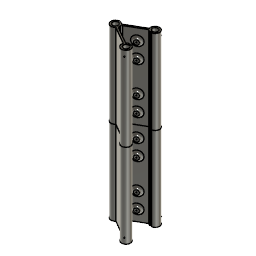
casomira-semafor-dlouhý (Autodesk Fusion 360 design; units mm, degrees)
Autodesk Fusion 360 part; units mm, degrees
other "Base Mesh Feature1" in component "part_object_id_3"
other "Base Mesh Feature1'" in component "part_object_id_2"
other "Base Mesh Feature1''" in component "part_object_id_1"
sketch "Sketch1" plane through (0, 0, 0) normal (0, 0, 1) x (1, 0, 0)
  circle A0 centre (69.45, 162.2) radius 5
  arc A1 (69.4, 161.6) -> (69.6, 161.6) centre (69.5, 162.4) ccw
  arc A2 (69.4, 161.6) -> (69.6, 161.6) centre (69.5, 162.3) ccw
  circle A3 centre (114.45, 188.2) radius 5
  circle A4 centre (114.45, 136.2003) radius 5
  line L0 (115.95, 142.25) -> (115.95, 182.2)
  line L1 (106.8955, 185.5676) -> (75.5037, 167.43)
  line L2 (75.5037, 156.97) -> (109.5697, 137.2876)
  line L3 (112.95, 142.25) -> (112.95, 182.2)
  line L4 (108.3963, 182.97) -> (77.0045, 164.8324)
  line L5 (77.0045, 159.5676) -> (108.3963, 141.4303)
  arc A5 (75.5037, 167.43) -> (75.5037, 156.97) centre (69.45, 162.2) ccw
  arc A6 (77.0045, 159.5676) -> (77.0045, 164.8324) centre (69.45, 162.2) ccw
  line L6 (114.45, 182.2) -> (112.95, 182.2)
  line L7 (114.45, 182.2) -> (115.95, 182.2)
  line L8 (114.45, 142.25) -> (112.95, 142.25)
  line L9 (114.45, 142.25) -> (115.95, 142.25)
  arc A7 (108.3963, 182.97) -> (112.95, 180.3419) centre (114.45, 188.2) ccw
  arc A8 (115.95, 180.3419) -> (106.8955, 185.5676) centre (114.45, 188.2) ccw
  arc A9 (106.8955, 138.8327) -> (115.95, 144.0584) centre (114.45, 136.2003) ccw
  arc A10 (112.95, 144.0584) -> (108.3963, 141.4303) centre (114.45, 136.2003) ccw
  line L10 (115.95, 182.2) -> (112.95, 182.2)
  line L11 (112.95, 182.2) -> (112.95, 142.25)
  line L12 (112.95, 142.25) -> (115.95, 142.25)
  line L13 (115.95, 142.25) -> (115.95, 182.2)
  dimension "d1" = 10
  dimension "d2" = 16
  dimension "d3" = 10
  dimension "d4" = 16
  dimension "d5" = 51.971
  dimension "d6" = 10
  dimension "d7" = 16
  constraint concentric A0 A5
  constraint concentric A3 A7
  constraint concentric A4 A9
  constraint concentric A5 A6
  constraint coincident A4 L2.end
  constraint perpendicular L3 L6
  constraint perpendicular L0 L7
  constraint perpendicular L3 L8
  constraint perpendicular L0 L9
  constraint coincident L2 A9.start
  constraint coincident L0 A8.start
  constraint concentric A7 A8
  constraint coincident L3 A7.end
  constraint coincident L0 A9.end
  constraint concentric A9 A10
  constraint coincident L3 A10.start
  constraint horizontal L10
  constraint vertical L11
  constraint horizontal L12
  constraint vertical L13
  measures "d1" diameter of A0
  measures "d2" diameter of A5
  measures "d3" diameter of A3
  measures "d4" diameter of A7
  measures "d5" distance of A0.centre A4.centre
  measures "d6" diameter of A4
  measures "d7" diameter of A9
sketch "Sketch2" plane through (0, 0, 0) normal (0, 1, 0) x (1, 0, 0)
extrude "Extrude1" add sketch "Sketch1" along normal blind 150 contours L0 L1 L2 L3 L4 L5 A5 A6 L6 L7 L8 L9 A7 A8 A9 A10 L10 L11 L12 L13 makes body 1
sketch "Sketch3" plane through (0, 0, 150) normal (0, 0, 1) x (-1, 0, 0)
  circle A0 centre (-114.45, -136.2003) radius 5
  circle A1 centre (-69.45, -162.2) radius 5
  circle A2 centre (-114.45, -188.2) radius 5
  arc A3 (-112.95, -144.0584) -> (-108.3963, -141.4303) centre (-114.45, -136.2003) ccw
  line L0 (-108.3963, -141.4303) -> (-77.0045, -159.5676)
  arc A4 (-77.0045, -159.5676) -> (-77.0045, -164.8324) centre (-69.45, -162.2) ccw
  line L1 (-77.0045, -164.8324) -> (-108.3963, -182.97)
  arc A5 (-108.3963, -182.97) -> (-112.95, -180.3419) centre (-114.45, -188.2) ccw
  line L2 (-112.95, -180.3419) -> (-112.95, -182.2)
  line L3 (-112.95, -182.2) -> (-115.95, -182.2)
  line L4 (-115.95, -182.2) -> (-115.95, -180.3419)
  arc A6 (-115.95, -180.3419) -> (-106.8955, -185.5676) centre (-114.45, -188.2) ccw
  line L5 (-106.8955, -185.5676) -> (-75.5037, -167.43)
  arc A7 (-75.5037, -167.43) -> (-75.5037, -156.97) centre (-69.45, -162.2) ccw
  line L6 (-75.5037, -156.97) -> (-106.8955, -138.8327)
  arc A8 (-106.8955, -138.8327) -> (-115.95, -144.0584) centre (-114.45, -136.2003) ccw
  line L7 (-115.95, -144.0584) -> (-115.95, -142.25)
  line L8 (-115.95, -142.25) -> (-112.95, -142.25)
  line L9 (-112.95, -142.25) -> (-112.95, -144.0584)
  line L10 (-69.45, -162.2) -> (-114.45, -136.2003)
  line L11 (-114.45, -136.2003) -> (-91.95, -149.2001)
  line L12 (-91.95, -149.2001) -> (-114.45, -188.2)
  line L13 (-114.45, -188.2) -> (-69.45, -162.2)
  line L14 (-91.95, -175.2) -> (-114.45, -136.2003)
  line L15 (-114.45, -136.2003) -> (-114.45, -188.2)
  constraint coincident A1.centre A4.centre
  constraint coincident A0.centre A3.centre
  constraint midpoint L10 L11.end
  constraint coincident A2.centre A5.centre
  constraint midpoint L13 L14.start
sketch "Sketch4" plane through (0, 0, 0) normal (0, 1, 0) x (1, 0, 0)
sketch "Sketch5" plane through (0, 0, 150) normal (0, 0, 1) x (-1, 0, 0)
sketch "Sketch6" plane through (0, 0, 150) normal (0, 0, 1) x (-1, 0, 0)
  line L0 (-91.95, -175.2) -> (-114.45, -136.2)
  line L1 (-114.45, -136.2) -> (-120.8561, -125.0961)
  line L2 (-91.95, -149.2) -> (-114.45, -188.2)
  line L3 (-114.45, -188.2) -> (-120.7, -199.0334)
  line L4 (-114.45, -188.2) -> (-114.45, -136.2)
  line L5 (-114.45, -162.2) -> (-69.45, -162.2)
  line L6 (-69.45, -162.2) -> (-57, -162.2)
  dimension "d13" = 180
  constraint parallel L2 L3
  constraint vertical L4
  constraint midpoint L4 L5.start
  constraint perpendicular L4 L5
  constraint parallel L5 L6
  measures "d13" angle of L0 L1
sketch "Sketch7" plane through (0, 0, 150) normal (0, 0, 1) x (-1, 0, 0)
  line L0 (-91.95, -149.2) -> (-120.7638, -199.107)
  line L1 (-91.95, -149.2) -> (-34.3224, -149.2) construction
  line L2 (-120.7638, -199.107) -> (-122.4959, -198.107)
  line L3 (-122.4959, -198.107) -> (-119.0318, -200.107)
  line L4 (-119.0318, -200.107) -> (-121.0318, -203.5711)
  line L5 (-121.0318, -203.5711) -> (-124.4959, -201.5711)
  line L6 (-124.4959, -201.5711) -> (-122.4959, -198.107)
  line L7 (-91.95, -175.2) -> (-120.9403, -124.9873)
  line L8 (-91.95, -175.2) -> (-33.9694, -175.2) construction
  line L9 (-120.9403, -124.9873) -> (-122.6724, -125.9873)
  line L10 (-122.6724, -125.9873) -> (-124.6724, -122.5232)
  line L11 (-124.6724, -122.5232) -> (-121.2083, -120.5232)
  line L12 (-121.2083, -120.5232) -> (-119.2083, -123.9873)
  line L13 (-119.2083, -123.9873) -> (-120.9403, -124.9873)
  line L14 (-57, -162.2) -> (-57, -164.2)
  line L15 (-57, -164.2) -> (-53, -164.2)
  line L16 (-53, -164.2) -> (-53, -160.2)
  line L17 (-53, -160.2) -> (-57, -160.2)
  line L18 (-57, -160.2) -> (-57, -162.2)
  dimension "d14" = 120
  dimension "d15" = 2
  dimension "d16" = 4
  dimension "d17" = 4
  dimension "d18" = 4
  dimension "d19" = 120
  dimension "d20" = 2
  dimension "d21" = 4
  dimension "d22" = 4
  dimension "d23" = 4
  dimension "d24" = 2
  dimension "d25" = 4
  dimension "d26" = 4
  constraint horizontal L1
  constraint perpendicular L0 L2
  constraint perpendicular L0 L3
  constraint perpendicular L3 L4
  constraint perpendicular L0 L5
  constraint horizontal L8
  constraint perpendicular L7 L9
  constraint perpendicular L9 L10
  constraint perpendicular L7 L11
  constraint perpendicular L9 L12
  constraint vertical L14
  constraint perpendicular L14 L15
  constraint perpendicular L15 L16
  constraint perpendicular L14 L17
  constraint perpendicular L17 L18
  measures "d14" angle of L0 L1
  measures "d15" distance of L0.end L2.end
  measures "d16" distance of L2.end L3.end
  measures "d17" distance of L3.end L4.end
  measures "d18" distance of L4.end L5.end
  measures "d19" angle of L7 L8
  measures "d20" distance of L7.end L9.end
  measures "d21" distance of L9.end L10.end
  measures "d22" distance of L10.end L11.end
  measures "d23" distance of L11.end L12.end
  measures "d24" distance of L14.start L14.end
  measures "d25" distance of L14.end L15.end
  measures "d26" distance of L15.end L16.end
extrude "Extrude2" add sketch "Sketch7" against normal blind 150 separate body makes body 2 at (120.5416, 121.6779, 100) makes body 3 at (119.6984, 201.2617, 100) makes body 4 at (57, 161.5333, 100)
sketch "Sketch8" plane through (-21.886, 37.9077, 0) normal (0.5, -0.866025, 0) x (0.866025, 0.5, 0)
  line L0 (169.231, 150) -> (165.231, 150)
  line L1 (165.231, 150) -> (165.231, 0)
  line L2 (165.231, 0) -> (169.231, 0)
  line L3 (169.231, 0) -> (169.231, 150)
  line L4 (167.231, 150) -> (167.231, 140)
  line L5 (167.231, 0) -> (167.231, 10)
  circle A0 centre (167.231, 10) radius 0.9
  circle A1 centre (167.231, 140) radius 0.9
  dimension "d29" = 10
  dimension "d30" = 10
  dimension "d31" = 1.8
  dimension "d32" = 1.8
  constraint midpoint L0 L4.start
  constraint perpendicular L0 L4
  constraint midpoint L2 L5.start
  constraint perpendicular L2 L5
  constraint coincident L5.end A0.centre
  constraint coincident L4.end A1.centre
  measures "d29" distance of L4.start L4.end
  measures "d30" distance of L5.start L5.end
  measures "d31" diameter of A0
  measures "d32" diameter of A1
extrude "Extrude3" cut sketch "Sketch8" against normal blind 20 contours A0 | A1 bodies 1 2
sketch "Sketch9" plane through (-52.1284, 90.2223, 0) normal (0.500278, -0.865865, 0) x (0.865865, 0.500278, 0)
  line L0 (149.1375, 0) -> (185.3924, 0)
  line L1 (185.3924, 0) -> (185.3924, 150)
  line L2 (185.3924, 150) -> (149.1375, 150)
  line L3 (149.1375, 150) -> (149.1375, 0)
sketch "Sketch10" plane through (53, 0, 0) normal (-1, 0, 0) x (0, -1, 0)
  line L0 (-160.2, 150) -> (-164.2, 150)
  line L1 (-164.2, 150) -> (-164.2, 0)
  line L2 (-164.2, 0) -> (-160.2, 0)
  line L3 (-160.2, 0) -> (-160.2, 150)
  line L4 (-162.2, 150) -> (-162.2, 140)
  line L5 (-162.2, 0) -> (-162.2, 10)
  circle A0 centre (-162.2, 10) radius 0.9
  circle A1 centre (-162.2, 140) radius 0.9
  dimension "d35" = 10
  dimension "d36" = 10
  dimension "d37" = 1.8
  dimension "d38" = 1.8
  constraint midpoint L0 L4.start
  constraint perpendicular L0 L4
  constraint midpoint L2 L5.start
  constraint perpendicular L2 L5
  constraint coincident L5.end A0.centre
  constraint coincident L4.end A1.centre
  measures "d35" distance of L4.start L4.end
  measures "d36" distance of L5.start L5.end
  measures "d37" diameter of A0
  measures "d38" diameter of A1
extrude "Extrude4" cut sketch "Sketch10" against normal blind 14 contours A0 | A1 bodies 1 4
sketch "Sketch11" plane through (118.4068, 205.0866, 0) normal (0.5, 0.866025, 0) x (-0.866025, 0.5, 0)
  line L0 (-3.031, 150) -> (-7.031, 150)
  line L1 (-7.031, 150) -> (-7.031, 0)
  line L2 (-7.031, 0) -> (-3.031, 0)
  line L3 (-3.031, 0) -> (-3.031, 150)
  line L4 (-5.031, 150) -> (-5.031, 140)
  line L5 (-5.031, 0) -> (-5.031, 10)
  circle A0 centre (-5.031, 10) radius 0.9
  circle A1 centre (-5.031, 140) radius 0.9
  dimension "d41" = 10
  dimension "d42" = 10
  dimension "d43" = 1.8
  dimension "d44" = 1.8
  constraint midpoint L0 L4.start
  constraint perpendicular L0 L4
  constraint midpoint L2 L5.start
  constraint perpendicular L2 L5
  constraint coincident L5.end A0.centre
  constraint coincident L4.end A1.centre
  measures "d41" distance of L4.start L4.end
  measures "d42" distance of L5.start L5.end
  measures "d43" diameter of A0
  measures "d44" diameter of A1
extrude "Extrude5" cut sketch "Sketch11" against normal blind 15 contours A0 | A1 bodies 1 3
extrude "Extrude6" cut 3 faces at (121.6963, 122.3446, 150) (55.6667, 161.5333, 150) (121.5198, 201.7497, 150) along direction (0, 0, -1) blind 210 on bodies 2 3 4 bodies 2 3 4
sketch "Sketch12" plane through (0, 0, 0) normal (0, 0, -1) x (1, 0, 0)
  circle A0 centre (114.45, -136.2003) radius 5
  circle A1 centre (69.45, -162.2) radius 5
  circle A2 centre (114.45, -188.2) radius 5
  arc A3 (108.3963, -141.4303) -> (112.95, -144.0584) centre (114.45, -136.2003) ccw
  line L0 (112.95, -144.0584) -> (112.95, -142.25)
  line L1 (112.95, -142.25) -> (115.95, -142.25)
  line L2 (115.95, -142.25) -> (115.95, -144.0584)
  arc A4 (115.95, -144.0584) -> (106.8955, -138.8327) centre (114.45, -136.2003) ccw
  line L3 (106.8955, -138.8327) -> (75.5037, -156.97)
  arc A5 (75.5037, -156.97) -> (75.5037, -167.43) centre (69.45, -162.2) ccw
  line L4 (75.5037, -167.43) -> (106.8955, -185.5676)
  arc A6 (106.8955, -185.5676) -> (115.95, -180.3419) centre (114.45, -188.2) ccw
  line L5 (115.95, -180.3419) -> (115.95, -182.2)
  line L6 (115.95, -182.2) -> (112.95, -182.2)
  line L7 (112.95, -182.2) -> (112.95, -180.3419)
  arc A7 (112.95, -180.3419) -> (108.3963, -182.97) centre (114.45, -188.2) ccw
  line L8 (108.3963, -182.97) -> (77.0045, -164.8324)
  arc A8 (77.0045, -164.8324) -> (77.0045, -159.5676) centre (69.45, -162.2) ccw
  line L9 (77.0045, -159.5676) -> (108.3963, -141.4303)
  line L10 (108.3963, -141.4303) -> (106.8955, -138.8327)
  line L11 (106.8955, -138.8327) -> (75.5037, -156.97)
  line L12 (75.5037, -156.97) -> (77.0045, -159.5676)
  line L13 (77.0045, -159.5676) -> (108.3963, -141.4303)
  constraint coincident A3.start L9.end
  constraint coincident A4.end L3.start
  constraint perpendicular L10 L11
  constraint coincident A8.end L9.start
  constraint perpendicular L9 L12
extrude "Extrude7" cut sketch "Sketch12" against normal blind 130 contours L3 L9 L10 L11 L12 L13 bodies 1
sketch "Sketch13" plane through (-52.1284, 90.2223, 0) normal (0.500278, -0.865865, 0) x (0.865865, 0.500278, 0)
  line L0 (185.39, 0) -> (149.15, 0)
  line L1 (149.15, 0) -> (167.27, 0)
  line L2 (167.27, 0) -> (167.27, 20)
  line L3 (185.39, 0) -> (149, 0)
  line L4 (149, 0) -> (149, 150)
  line L5 (149, 150) -> (185.39, 150)
  line L6 (185.39, 150) -> (185.39, 0)
  line L7 (167.195, 150) -> (167.195, 130)
  line L8 (167.195, 130) -> (170.195, 130)
  line L9 (170.195, 130) -> (170.195, 102)
  line L10 (167.27, 20) -> (170.27, 20)
  line L11 (170.27, 20) -> (170.27, 48)
  circle A0 centre (170.27, 20) radius 0.9
  circle A1 centre (170.27, 48) radius 0.9
  circle A2 centre (170.195, 102) radius 0.9
  circle A3 centre (170.195, 130) radius 0.9
  circle A4 centre (170.195, 130) radius 4
  circle A5 centre (170.195, 102) radius 4
  circle A6 centre (170.27, 48) radius 4
  circle A7 centre (170.27, 20) radius 4
  dimension "d51" = 20
  dimension "d52" = 20
  dimension "d53" = 3
  dimension "d54" = 28
  dimension "d55" = 3
  dimension "d56" = 28
  dimension "d57" = 1.8
  dimension "d58" = 1.8
  dimension "d59" = 1.8
  dimension "d60" = 1.8
  dimension "d61" = 8
  dimension "d62" = 8
  dimension "d63" = 8
  dimension "d64" = 8
  constraint horizontal L0
  constraint midpoint L0 L1.end
  constraint perpendicular L0 L2
  constraint horizontal L3
  constraint vertical L4
  constraint horizontal L5
  constraint vertical L6
  constraint midpoint L5 L7.start
  constraint perpendicular L5 L7
  constraint perpendicular L7 L8
  constraint perpendicular L8 L9
  constraint perpendicular L2 L10
  constraint perpendicular L10 L11
  constraint coincident L10.end L11.start
  constraint coincident L11.end A1.centre
  constraint coincident L9.end A2.centre
  constraint coincident L8.end L9.start
  constraint concentric A3 A4
  measures "d51" distance of L1.end L2.end
  measures "d52" distance of L7.start L7.end
  measures "d53" distance of L7.end L8.end
  measures "d54" distance of L8.end L9.end
  measures "d55" distance of L2.end L10.end
  measures "d56" distance of L10.end L11.end
  measures "d57" diameter of A0
  measures "d58" diameter of A1
  measures "d59" diameter of A2
  measures "d60" diameter of A3
  measures "d61" diameter of A4
  measures "d62" diameter of A5
  measures "d63" diameter of A6
  measures "d64" diameter of A7
extrude "Extrude8" add sketch "Sketch13" along normal blind 5 contours L2 L10 L11 A0 A7 | L2 L10 L11 A0 A7 | L7 L8 L9 A3 A4 | L7 L8 L9 A3 A4 | A5 | A6 bodies 1 2 3 4
extrude "Extrude9" cut 4 faces at (97.0302, 170.6283, 17.1797) (98.5403, 171.5008, 45.1665) (96.3119, 170.2133, 104.457) (95.3615, 169.6641, 131.1017) along direction (-0.500278, 0.865865, 0) blind 1 on bodies 1 bodies 1
fillet "Fillet1" radius 5 4 edges at (92.0733, 173.5389, 21.4465) (92.0733, 173.5389, 49.4465) (92.0084, 173.5014, 103.4465) (92.0084, 173.5014, 131.4465) on bodies 1
extrude "Extrude10" add 1 faces at (86.9682, 152.656, 130) along direction (0, 0, -1) blind 130 on bodies 1 bodies 1
sketch "Sketch14" plane through (0, 0, 150) normal (0, 0, 1) x (-1, 0, 0)
  line L0 (-70, -162.2) -> (-80, -162.2)
  line L1 (-80, -162.2) -> (-80, -164)
  line L2 (-80, -164) -> (-80, -160)
  line L3 (-83, -160) -> (-83, -164)
  line L4 (-80, -160) -> (-80, -164.813)
  line L5 (-80, -164.813) -> (-83, -164.813)
  line L6 (-83, -164.813) -> (-83, -160)
  line L7 (-80, -160) -> (-80, -159.6103)
  line L8 (-80, -159.6103) -> (-83, -159.6103)
  line L9 (-83, -159.6103) -> (-83, -160)
  line L10 (-114.45, -162.2) -> (-83, -162.2)
  line L11 (-80, -162.2) -> (-70, -162.2)
  constraint horizontal L10
  constraint perpendicular L1 L11
  constraint perpendicular L2 L11
  constraint perpendicular L4 L11
  constraint perpendicular L2 L5
  constraint perpendicular L7 L8
  constraint coincident L3 L10.end
  constraint collinear L10 L11
extrude "Extrude11" add sketch "Sketch14" against normal blind 130 separate body makes body 5
extrude "Extrude12" cut 1 faces at (82, 160.7333, 150) along direction (0, 0, -1) blind 20 on bodies 5 bodies 5
extrude "Extrude13" cut 1 faces at (83, 163.0788, 93.3333) along direction (-1, 0, 0) blind 15 on bodies 5 bodies 1 5
fillet "Fillet2" radius 2.5 2 edges at (77.0045, 159.5676, 75) (77.0045, 164.8324, 75) on bodies 1
fillet "Fillet3" radius 2.6 4 edges at (75.6939, 164.813, 20) (75.6945, 159.6103, 20) (75.6939, 164.813, 130) (75.6945, 159.6103, 130) on bodies 1
sketch "Sketch15" plane through (0, 0, 150) normal (0, 0, 1) x (-1, 0, 0)
  circle A0 centre (-114.45, -136.2003) radius 5
  circle A1 centre (-69.45, -162.2) radius 5
  circle A2 centre (-114.45, -188.2) radius 5
  arc A3 (-112.95, -144.0584) -> (-108.3963, -141.4303) centre (-114.45, -136.2003) ccw
  line L0 (-108.3963, -141.4303) -> (-78.6065, -158.642)
  arc A4 (-77.3793, -161.1384) -> (-78.6065, -158.642) centre (-79.8571, -160.8067) ccw
  arc A5 (-77.3793, -161.1384) -> (-77.3792, -163.2616) centre (-69.45, -162.2) ccw
  arc A6 (-78.6064, -165.758) -> (-77.3792, -163.2616) centre (-79.8571, -163.5934) ccw
  line L1 (-78.6064, -165.758) -> (-108.3963, -182.97)
  arc A7 (-108.3963, -182.97) -> (-112.95, -180.3419) centre (-114.45, -188.2) ccw
  line L2 (-112.95, -180.3419) -> (-112.95, -182.2)
  line L3 (-112.95, -182.2) -> (-115.95, -182.2)
  line L4 (-115.95, -182.2) -> (-115.95, -180.3419)
  arc A8 (-115.95, -180.3419) -> (-106.8955, -185.5676) centre (-114.45, -188.2) ccw
  line L5 (-106.8955, -185.5676) -> (-75.5037, -167.43)
  arc A9 (-75.5037, -167.43) -> (-75.5037, -156.97) centre (-69.45, -162.2) ccw
  line L6 (-75.5037, -156.97) -> (-106.8955, -138.8327)
  arc A10 (-106.8955, -138.8327) -> (-115.95, -144.0584) centre (-114.45, -136.2003) ccw
  line L7 (-115.95, -144.0584) -> (-115.95, -142.25)
  line L8 (-115.95, -142.25) -> (-112.95, -142.25)
  line L9 (-112.95, -142.25) -> (-112.95, -144.0584)
  circle A11 centre (-114.45, -188.2) radius 8
  circle A12 centre (-69.45, -162.2) radius 8
  circle A13 centre (-114.45, -136.2003) radius 8
  constraint concentric A2 A11
  constraint concentric A1 A12
  constraint concentric A0 A13
  constraint coincident L6.end A13
extrude "Extrude14" cut sketch "Sketch15" against normal blind 15 contours A3 A10 L7 L8 L9 A13 | A5 A9 A12 | A7 L2 L3 L4 A8 A11 bodies 1
extrude "Extrude15" add 3 faces at (62.4644, 162.2, 135) (117.0221, 182.3951, 135) (117.0221, 142.0217, 135) along direction (0, 0, 1) blind 15 on bodies 1 bodies 1 5
mirror "Mirror1" about plane through (0, 0, 150) normal (0, 0, 1) of bodies 1 makes body 6
component "CasomieraPart1_OnlyTruss" placed x (1, 0, 0) y (0, 1, 0) z (0, 0, 1) at (0, 0, 0)
component "part_object_id_3" placed x (1, 0, 0) y (0, 1, 0) z (0, 0, 1) at (0, 0, 0) in component "Component"
component "part_object_id_3" placed x (1, 0, 0) y (0, 1, 0) z (0, 0, 1) at (0, 0, 0) in component "Component'"
component "part_object_id_3" placed x (1, 0, 0) y (0, 1, 0) z (0, 0, 1) at (0, 0, 0) in component "Component''"
component "part_object_id_3" placed x (1, 0, 0) y (0, 1, 0) z (0, 0, 1) at (0, 0, 0) in component "Component'''"
component "part_object_id_2" placed x (1, 0, 0) y (0, 1, 0) z (0, 0, 1) at (0, 0, 0) in component "Component''''"
component "part_object_id_2" placed x (1, 0, 0) y (0, 1, 0) z (0, 0, 1) at (0, 0, 0) in component "Component'''''"
component "part_object_id_2" placed x (1, 0, 0) y (0, 1, 0) z (0, 0, 1) at (0, 0, 0) in component "Component''''''"
component "part_object_id_2" placed x (1, 0, 0) y (0, 1, 0) z (0, 0, 1) at (0, 0, 0) in component "Component'''''''"
component "part_object_id_2" placed x (1, 0, 0) y (0, 1, 0) z (0, 0, 1) at (0, 0, 0) in component "Component''''''''"
component "part_object_id_2" placed x (1, 0, 0) y (0, 1, 0) z (0, 0, 1) at (0, 0, 0) in component "Component'''''''''"
component "part_object_id_2" placed x (1, 0, 0) y (0, 1, 0) z (0, 0, 1) at (0, 0, 0) in component "Component''''''''''"
component "part_object_id_2" placed x (1, 0, 0) y (0, 1, 0) z (0, 0, 1) at (0, 0, 0) in component "Component'''''''''''"
component "part_object_id_2" placed x (1, 0, 0) y (0, 1, 0) z (0, 0, 1) at (0, 0, 0) in component "Component''''''''''''"
component "part_object_id_1" placed x (1, 0, 0) y (0, 1, 0) z (0, 0, 1) at (0, 0, 0) in component "Component'''''''''''''"
component "part_object_id_1" placed x (1, 0, 0) y (0, 1, 0) z (0, 0, 1) at (0, 0, 0) in component "Component''''''''''''''"
component "part_object_id_1" placed x (1, 0, 0) y (0, 1, 0) z (0, 0, 1) at (0, 0, 0) in component "Component'''''''''''''''"
component "part_object_id_1" placed x (1, 0, 0) y (0, 1, 0) z (0, 0, 1) at (0, 0, 0) in component "Component''''''''''''''''"
component "part_object_id_1" placed x (1, 0, 0) y (0, 1, 0) z (0, 0, 1) at (0, 0, 0) in component "Component'''''''''''''''''"
component "part_object_id_1" placed x (1, 0, 0) y (0, 1, 0) z (0, 0, 1) at (0, 0, 0) in component "Component''''''''''''''''''"
component "part_object_id_1" placed x (1, 0, 0) y (0, 1, 0) z (0, 0, 1) at (0, 0, 0) in component "Component'''''''''''''''''''"
component "part_object_id_1" placed x (1, 0, 0) y (0, 1, 0) z (0, 0, 1) at (0, 0, 0) in component "Component''''''''''''''''''''"
component "part_object_id_1" placed x (1, 0, 0) y (0, 1, 0) z (0, 0, 1) at (0, 0, 0) in component "Component'''''''''''''''''''''"
component "Component" placed x (0.5, 0.866025, 0) y (-0.866025, 0.5, 0) z (0, 0, 1) at (164.6988, 168.7277, 75) in component "CasomieraPart1_OnlyTruss"
component "Component'" placed x (0.5, 0.866025, 0) y (-0.866025, 0.5, 0) z (0, 0, 1) at (103.2031, 168.7277, 75) in component "CasomieraPart1_OnlyTruss"
component "Component''" placed x (0.5, 0.866025, 0) y (-0.866025, 0.5, 0) z (0, 0, 1) at (164.6988, 100.2746, 75) in component "CasomieraPart1_OnlyTruss"
component "Component'''" placed x (0.5, 0.866025, 0) y (-0.866025, 0.5, 0) z (0, 0, 1) at (103.2031, 100.2747, 75) in component "CasomieraPart1_OnlyTruss"
component "Component''''" placed x (1, 0, 0) y (0, 1, 0) z (0, 0, 1) at (75.0685, 112.4913, 14.8563) in component "CasomieraPart1_OnlyTruss"
component "Component'''''" placed x (1, 0, 0) y (0, 1, 0) z (0, 0, 1) at (80.9866, 120.9136, 14.8563) in component "CasomieraPart1_OnlyTruss"
component "Component''''''" placed x (1, 0, 0) y (0, 1, 0) z (0, 0, 1) at (70.7314, 121.8354, 14.8563) in component "CasomieraPart1_OnlyTruss"
component "Component'''''''" placed x (1, 0, 0) y (0, 1, 0) z (0, 0, 1) at (65.9024, 107.8079, 14.8563) in component "CasomieraPart1_OnlyTruss"
component "Component''''''''" placed x (1, 0, 0) y (0, 1, 0) z (0, 0, 1) at (76.6495, 130.2576, 14.8563) in component "CasomieraPart1_OnlyTruss"
component "Component'''''''''" placed x (1, 0, 0) y (0, 1, 0) z (0, 0, 1) at (91.2395, 121.8276, 14.8563) in component "CasomieraPart1_OnlyTruss"
component "Component''''''''''" placed x (1, 0, 0) y (0, 1, 0) z (0, 0, 1) at (86.9024, 131.1717, 14.8563) in component "CasomieraPart1_OnlyTruss"
component "Component'''''''''''" placed x (1, 0, 0) y (0, 1, 0) z (0, 0, 1) at (66.3944, 131.1794, 14.8563) in component "CasomieraPart1_OnlyTruss"
component "Component''''''''''''" placed x (1, 0, 0) y (0, 1, 0) z (0, 0, 1) at (80.9788, 139.5998, 14.8563) in component "CasomieraPart1_OnlyTruss"
component "Component'''''''''''''" placed x (1, 0, 0) y (0, 1, 0) z (0, 0, 1) at (97.1631, 130.2524, 14.9502) in component "CasomieraPart1_OnlyTruss"
component "Component''''''''''''''" placed x (1, 0, 0) y (0, 1, 0) z (0, 0, 1) at (70.7189, 140.5266, 14.9502) in component "CasomieraPart1_OnlyTruss"
component "Component'''''''''''''''" placed x (1, 0, 0) y (0, 1, 0) z (0, 0, 1) at (66.3546, 80.098, 14.9502) in component "CasomieraPart1_OnlyTruss"
component "Component''''''''''''''''" placed x (1, 0, 0) y (0, 1, 0) z (0, 0, 1) at (125.0143, 128.0041, 14.9502) in component "CasomieraPart1_OnlyTruss"
component "Component'''''''''''''''''" placed x (1, 0, 0) y (0, 1, 0) z (0, 0, 1) at (127.8503, 118.1032, 14.9502) in component "CasomieraPart1_OnlyTruss"
component "Component''''''''''''''''''" placed x (1, 0, 0) y (0, 1, 0) z (0, 0, 1) at (127.8503, 137.9051, 14.9502) in component "CasomieraPart1_OnlyTruss"
component "Component'''''''''''''''''''" placed x (1, 0, 0) y (0, 1, 0) z (0, 0, 1) at (127.8503, 107.7981, 14.9502) in component "CasomieraPart1_OnlyTruss"
component "Component''''''''''''''''''''" placed x (1, 0, 0) y (0, 1, 0) z (0, 0, 1) at (75.2701, 74.9507, 14.9502) in component "CasomieraPart1_OnlyTruss"
component "Component'''''''''''''''''''''" placed x (1, 0, 0) y (0, 1, 0) z (0, 0, 1) at (135.0018, 125.5135, 14.9502) in component "CasomieraPart1_OnlyTruss"
